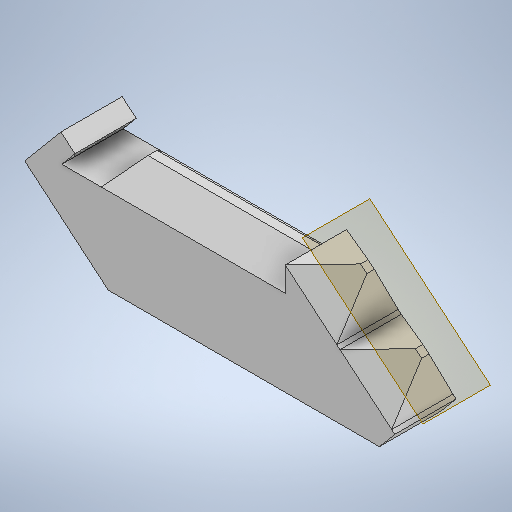
# Autodesk Inventor part: МОО 000 Пример емкости
Saved by Autodesk Inventor 2025 (Build 290162010, 162A)
## iProperties
Created: 2024-04-15
Part Number: МОО 000 Пример емкости
Material: Generic
Document SubType Name: Modeling
Designer: pokla
Density: 1 g/cm^3
Appearance: Default
Mass: 2.80856e+07 g
Surface Area: 700480 cm^2
Volume: 2.80856e+07 cm^3
Author: pokla
Autodesk Inventor part; units mm, degrees
ref_plane "YZ Plane" through (0, 0, 0) normal (1, 0, 0) x (0, 1, 0)
ref_plane "XZ Plane" through (0, 0, 0) normal (0, 1, 0) x (-1, 0, 0)
ref_plane "XY Plane" through (0, 0, 0) normal (0, 0, 1) x (1, 0, 0)
sketch "Sketch1" plane through (0, 0, 0) normal (0, 0, 1) x (1, 0, 0)
  line L0 (-3317.106, 0) -> (3317.106, 0)
  line L1 (3317.106, 0) -> (3694.4224, 449.6681)
  line L2 (3694.4224, 449.6681) -> (1013.2668, 2699.4247)
  line L3 (1013.2668, 2699.4247) -> (1013.2668, 2099.4247)
  line L4 (1013.2668, 2099.4247) -> (-4454.7332, 2099.4247)
  line L5 (-4454.7332, 2099.4247) -> (-4133.3394, 2482.4469)
  line L6 (-4133.3394, 2482.4469) -> (-4478.0594, 2771.7014)
  line L7 (-4478.0594, 2771.7014) -> (-5363.1779, 1716.8582)
  line L8 (-5363.1779, 1716.8582) -> (-3317.0732, -0.0275)
  point P0 (0, 0)
  point P1 (0, 0)
  dimension "d19" = 587
  dimension "d20" = 130
  dimension "d21" = 3500
  dimension "d22" = 90
  dimension "d28" = 600
  dimension "d29" = 50
  dimension "d30" = 5468
  dimension "d31" = 90
  dimension "d32" = 500
  dimension "d33" = 50
  dimension "d34" = 450
  dimension "d35" = 90
  dimension "d36" = 1377
  dimension "d37" = 90
  dimension "d38" = 2671
  dimension "d39" = 90
  dimension "d40" = 6634.2121
  dimension "d41" = 140
  constraints: 18 end point, 2 coincident, 1 horizontal, 1 midpoint, 1 point on line
  measures "d19" distance of L0.end L1.end
  measures "d20" angle of L0 L1
  measures "d21" distance of L1.end L2.end
  measures "d22" angle of L1 L2
  measures "d28" distance of L2.end L3.end
  measures "d29" angle of L2 L3
  measures "d30" distance of L3.end L4.end
  measures "d31" angle of L3 L4
  measures "d32" distance of L4.end L5.end
  measures "d33" angle of L5 L4
  measures "d34" distance of L5.end L6.end
  measures "d35" angle of L6 L5
  measures "d36" distance of L6.end L7.end
  measures "d37" angle of L6 L7
  measures "d38" distance of L7.end L8.end
  measures "d39" angle of L8 L7
  measures "d40" distance of L0.start L0.end
  measures "d41" angle of L8 L0
extrude "Extrusion1" add sketch "Sketch1" along normal mid plane 1500
sketch "Sketch2" plane through (1013.2668, 2699.4247, 750) normal (0.6428, 0.766, 0) x (0.766, -0.6428, 0)
  line L0 (3400, 0) -> (1750, 0)
  line L1 (1750, 0) -> (1750, 1500)
  line L2 (1750, 1500) -> (3400, 1500)
  line L3 (3400, 1500) -> (3400, 0)
  line L4 (0, 1500) -> (0, 0) projected
  line L5 (3500, 0) -> (0, 0) projected
  line L6 (3500, 1500) -> (3500, 0) projected
  line L7 (0, 1500) -> (3500, 1500) projected
  point P0 (958.9494, 750)
  point P1 (3400, 750)
  point P2 (3500, 750)
  dimension "d44" = 1650
  dimension "d45" = 1500
  dimension "d46" = 100
  constraints: 8 end point, 2 midpoint, 2 parallel, 1 horizontal, 1 horizontal alignment, 1 perpendicular
  measures "d44" distance of L1.end L2.end
  measures "d45" distance of L0.end L1.end
  measures "d46" distance between parallel lines of L6 L3
ref_plane "Work Plane1" through (1643.1987, 3450.1483, 750) normal (0.6428, 0.766, 0) x (0.766, -0.6428, 0)
sketch "Sketch3" plane through (1643.1987, 3450.1483, 750) normal (0.6428, 0.766, 0) x (0.766, -0.6428, 0)
  line L0 (1750, 0) -> (1750, 1500) construction
  line L1 (1750, 1500) -> (3400, 1500) construction
  line L2 (3400, 1500) -> (3400, 0) construction
  line L3 (3400, 0) -> (1750, 0) construction
  line L4 (1750, 750) -> (3400, 750) construction
  line L5 (2575, 0) -> (2575, 1500) construction
  line L6 (2475, 659) -> (2675, 659)
  line L7 (2675, 659) -> (2675, 841)
  line L8 (2675, 841) -> (2475, 841)
  line L9 (2475, 841) -> (2475, 659)
  line L10 (2475, 659) -> (2675, 841) construction
  point P0 (958.9494, 750)
  point P1 (2575, 750)
  dimension "d48" = 182
  dimension "d49" = 200
  constraints: 14 end point, 6 midpoint, 2 parallel, 1 horizontal, 1 perpendicular
  measures "d48" distance of L8.end L6.start
  measures "d49" distance of L6.start L6.end
loft "Loft1" add profiles "Sketch3", "Sketch2" contours all / L0 L1 L2 L3
sketch "Sketch4" plane through (1013.2668, 2699.4247, 750) normal (0.6428, 0.766, 0) x (0.766, -0.6428, 0)
  line L0 (0, 0) -> (1650, 0)
  line L1 (1650, 0) -> (1650, 1500)
  line L2 (1650, 1500) -> (0, 1500)
  line L3 (0, 1500) -> (0, 0)
  line L4 (1750, 0) -> (1750, 1500) projected
  line L5 (0, 1500) -> (1750, 1500) projected
  line L6 (0, 1500) -> (0, 0) projected
  line L7 (1750, 0) -> (0, 0) projected
  point P0 (958.9494, 750)
  point P1 (1650, 750)
  point P2 (1750, 750)
  dimension "d54" = 1650
  dimension "d55" = 1500
  dimension "d56" = 100
  constraints: 8 end point, 2 midpoint, 2 parallel, 1 horizontal, 1 horizontal alignment, 1 perpendicular
  measures "d54" distance of L2.end L1.end
  measures "d55" distance of L1.end L0.end
  measures "d56" distance between parallel lines of L4 L1
sketch "Sketch5" plane through (1643.1987, 3450.1483, 750) normal (0.6428, 0.766, 0) x (0.766, -0.6428, 0)
  line L0 (0, 1500) -> (1750, 1500) construction
  line L1 (0, 1500) -> (0, 0) construction
  line L2 (1650, 0) -> (1650, 1500) construction
  line L3 (0, 0) -> (1650, 0) construction
  line L4 (1650, 0) -> (0, 1500) construction
  line L5 (0, 0) -> (1650, 1500) construction
  line L6 (725, 659) -> (925, 659)
  line L7 (925, 659) -> (925, 841)
  line L8 (925, 841) -> (725, 841)
  line L9 (725, 841) -> (725, 659)
  line L10 (925, 659) -> (725, 841) construction
  point P0 (958.9494, 750)
  point P1 (825, 750)
  dimension "d59" = 200
  dimension "d60" = 182
  constraints: 14 end point, 2 midpoint, 2 parallel, 1 horizontal, 1 perpendicular
  measures "d59" distance of L8.end L7.end
  measures "d60" distance of L8.end L6.start
loft "Loft2" add profiles "Sketch5", "Sketch4" contours all / L3 L2 L1 L0
sketch "Sketch6" plane through (1013.2668, 2099.4247, -750) normal (-1, 0, 0) x (0, 0, 1)
  line L0 (0, 0) -> (1500, 0) projected
  line L1 (0, 0) -> (0, 600) projected
  line L2 (0, 600) -> (1500, 600) projected
  line L3 (1500, 600) -> (1500, 0) projected
  line L4 (860, 600) -> (640, 600)
  line L5 (1500, 0) -> (0, 0)
  line L6 (860, 600) -> (1500, 0)
  line L7 (640, 600) -> (0, 0)
  point P0 (750, -2099.4247)
  point P1 (750, 600)
  point P2 (640, 600)
  point P3 (860, 600)
  dimension "d65" = 220
  constraints: 8 end point, 2 midpoint, 1 collinear, 1 horizontal
  measures "d65" distance of L4.start L4.end
extrude "Extrusion2" add sketch "Sketch6" along normal blind 4500 contours L7 L2 L6 L0
sketch "Sketch7" plane through (-3486.7332, 2099.4247, -750) normal (-1, 0, 0) x (0, 0, 1)
  point P0 (750, -2099.4247)
sketch "Sketch8" plane through (0, 0, 750) normal (0, 0, 1) x (1, 0, 0)
  line L0 (1013.2668, 2699.4247) -> (1013.2668, 2099.4247) projected
  line L1 (1013.2668, 2699.4247) -> (-3486.7332, 2699.4247) projected
  line L2 (-3486.7332, 2099.4247) -> (-3486.7332, 2699.4247) projected
  line L3 (1013.2668, 2099.4247) -> (-3486.7332, 2099.4247) projected
  line L4 (-3486.7332, 2099.4247) -> (-2986.7722, 2699.4247)
  point P0 (0, 0)
  dimension "d69" = 781
  constraints: 2 end point, 1 point on line
  measures "d69" distance of L2.start L4.end
extrude "Extrusion3" cut sketch "Sketch8" against normal through all contours L4 L2 L1
body "Solid1"
